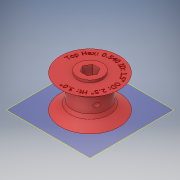
# Autodesk Inventor part: spoolV08upper
Saved by Autodesk Inventor 2019.4 (Build 234330000, 330)
## iProperties
Created: 2019-02-25
Part Number: spoolV08upper
Material: PC/ABS Plastic
Document SubType Name: Modeling
Designer: steele
Density: 0.357273 g/cm^3
Appearance: Smooth - Red
holeForString: 0.200 in
stringDiameter: 0.120 in
clearanceForString: 0.080 in
clearanceForHexShaft: 0.040 in
spoolInteriorDiameter: 1.500 in
spoolInteriroRadius: 0.750 in
spoolExteriorDiameter: 2.500 in
spoolExteriorRadius: 1.250 in
hexHoleChamfer: 0.063 in
stringHoleCenterFromHexShaft: 0.370 in
textCircleDiameter: 1.875 in
textHeight: 0.180 in
textDepth: 0.050 in
Author: steele
Autodesk Inventor part; units mm, degrees
(part 1 of 2)
ref_plane "XZ Plane" through (0, 0, 0) normal (0, 1, 0) x (-1, 0, 0)
sketch "Sketch15" plane through (0, 0, 0) normal (0, 0, 1) x (1, 0, 0)
  line L0 (31.75, 0) -> (31.75, 69.85) construction
  line L1 (12.065, 0) -> (31.75, 0)
  line L2 (13.335, 69.85) -> (31.75, 69.85)
  line L3 (19.05, 0) -> (19.05, 69.85) construction
  line L4 (0, 69.85) -> (0, 0)
  line L5 (19.05, 17.4625) -> (31.75, 17.4625) construction
  line L6 (31.75, 0) -> (19.05, 7.3323)
  line L7 (31.75, 34.925) -> (19.05, 27.5927)
  line L8 (19.05, 27.5927) -> (31.75, 27.5927) construction
  line L9 (19.05, 27.5927) -> (19.05, 7.3323)
  line L10 (31.75, 34.925) -> (19.05, 42.2573)
  line L11 (19.05, 42.2573) -> (19.05, 62.5177)
  line L12 (19.05, 62.5177) -> (31.75, 69.85)
  line L13 (31.75, 34.925) -> (19.05, 34.925) construction
  line L14 (19.05, 62.5177) -> (31.75, 62.5177) construction
  line L15 (0, 69.85) -> (0, 72.39)
  line L16 (0, 72.39) -> (13.335, 72.39)
  line L17 (13.335, 72.39) -> (13.335, 69.85)
  line L18 (0, 0) -> (0, -2.54)
  line L19 (0, -2.54) -> (12.065, -2.54)
  line L20 (12.065, -2.54) -> (12.065, 0)
  dimension "d85" = 31.75
  dimension "d86" = 69.85
  dimension "d87" = 19.05
  dimension "d88" = 31.75
  dimension "d89" = 34.925
  dimension "centerLineForSpool" = 17.4625
  dimension "d93" = 30
  dimension "d94" = 30
  dimension "d95" = 30
  dimension "d96" = 30
  dimension "d149" = 2.54
  dimension "d150" = 13.335
  dimension "d151" = 2.54
  dimension "d152" = 12.065
  constraints: 42 end point, 10 point on line, 5 perpendicular, 3 horizontal, 3 vertical, 2 midpoint, 1 collinear, 1 parallel
  measures "d85" distance from line of L4.end L0
  measures "d86" distance of L0.start L0.end
  measures "d87" distance from line of L3 L4.end
  measures "d88" distance of L4.start L0.end
  measures "d89" distance from line of L7.start L1
  measures "centerLineForSpool" distance from line of L5.start L1
  measures "d93" angle of L6 L1
  measures "d94" angle of L7 L8
  measures "d95" angle of L10 L13
  measures "d96" angle of L12 L14
  measures "d149" distance between parallel lines of L16 L2
  measures "d150" distance between parallel lines of L17 L15
  measures "d151" distance from line of L4.end L19
  measures "d152" distance between parallel lines of L20 L18
revolve "Revolution2" add sketch "Sketch15" angle 360 about axis through (0, 69.85, 0) along (0, -1, 0)
sketch "Sketch16" plane through (0, 0, 0) normal (0, -1, 0) x (1, 0, 0)
  line L0 (-7.9189, 0) -> (-3.9595, 6.858)
  line L1 (-3.9595, 6.858) -> (3.9595, 6.858)
  line L2 (3.9595, 6.858) -> (7.9189, 0)
  line L3 (7.9189, 0) -> (3.9595, -6.858)
  line L4 (3.9595, -6.858) -> (-3.9595, -6.858)
  line L5 (-3.9595, -6.858) -> (-7.9189, 0)
  point P0 (0, 0)
  point P1 (0, 0)
  dimension "d103" = 13.716
  constraints: 12 end point, 1 coincident, 1 horizontal, 13 other
  measures "d103" distance between parallel lines of L1 L4
extrude "Extrusion11" cut sketch "Sketch16" against normal through all
sketch "Sketch17" plane through (0, 0, 0) normal (1, 0, 0) x (0, 1, 0)
  circle A0 centre (52.3875, 9.398) radius 2.54
  circle A1 centre (17.4625, 9.398) radius 2.54
  line L0 (0, 31.75) -> (0, -31.75) projected
  line L1 (69.85, 31.75) -> (69.85, -31.75) projected
  line L2 (0, 6.858) -> (72.39, 6.858) projected
  point P0 (0, 0)
  point P1 (69.85, 6.858)
  dimension "d110" = 17.4625
  dimension "d111" = 17.4625
  dimension "d112" = 5.08
  constraints: 2 centre point, 2 tangent, 1 equal radius
  measures "d110" distance from line of A1.centre L0
  measures "d111" distance from line of A0.centre L1
  measures "d112" diameter of A0
extrude "Extrusion13" cut sketch "Sketch17" along normal through all both and the other way through all
ref_plane "Work Plane4" through (-19.05, 0, 0) normal (1, 0, 0) x (0, 1, 0)
sketch "Sketch22" plane through (-19.05, 0, 0) normal (1, 0, 0) x (0, 1, 0)
  spline S0 degree 7 poles (54.9275, 9.398) (54.9275, 9.7003) (54.8855, 9.9947) (54.8055, 10.2759) (54.6914, 10.5396) (54.547, 10.7823) (54.3764, 11.0012) (53.983, 11.3946) (53.7559, 11.5694) (53.5066, 11.7139) (53.24, 11.8248) (52.9612, 11.9) (52.6753, 11.938) (52.1137, 11.938) (51.8403, 11.9036) (51.5721, 11.8349) (51.3141, 11.7328) (51.0711, 11.5991) (50.848, 11.4367) (50.4419, 11.0554) (50.2585, 10.8324) (50.103, 10.5833) (49.9797, 10.311) (49.8931, 10.0193) (49.8475, 9.713) (49.8475, 9.1243) (49.8819, 8.8508) (49.9506, 8.5825) (50.0528, 8.3245) (50.1864, 8.0817) (50.3487, 7.8586) (50.7502, 7.431) (50.9916, 7.2397) (51.2531, 7.0865) (51.5286, 6.9719) (51.8128, 6.8958) (52.1007, 6.858) (52.7051, 6.858) (53.0247, 6.9043) (53.3394, 6.998) (53.642, 7.1395) (53.9245, 7.3282) (54.1787, 7.563) (54.5393, 8.0279) (54.6661, 8.2331) (54.7705, 8.4538) (54.8497, 8.6855) (54.9021, 8.9235) (54.9275, 9.1626) (54.9275, 9.398) knots 0 0 0 0 0 0 0 0 0.127217 0.127217 0.127217 0.127217 0.127217 0.127217 0.25952 0.25952 0.25952 0.25952 0.25952 0.25952 0.385403 0.385403 0.385403 0.385403 0.385403 0.385403 0.516079 0.516079 0.516079 0.516079 0.516079 0.516079 0.629606 0.629606 0.629606 0.629606 0.629606 0.629606 0.75956 0.75956 0.75956 0.75956 0.75956 0.75956 0.903464 0.903464 0.903464 0.903464 0.903464 0.903464 1 1 1 1 1 1 1 1 projected
  circle A0 centre (52.3875, 9.398) radius 4.7625
  circle A1 centre (52.3875, 9.398) radius 2.54 construction
  line L0 (52.3875, 6.858) -> (72.39, 6.858) construction
  line L1 (69.85, 31.75) -> (69.85, -31.75) construction
  point P0 (0, 0)
  point P1 (69.85, 6.858)
  dimension "d121" = 17.4625
  dimension "d122" = 5.08
  dimension "d125" = 9.525
  constraints: 2 centre point, 1 concentric, 1 tangent, 1 vertical alignment
  measures "d121" distance from line of A1.centre L1
  measures "d122" diameter of A1
  measures "d125" diameter of A0
extrude "Extrusion16" cut sketch "Sketch22" along normal blind 11.1125
ref_plane "Work Plane5" through (19.05, 0, 0) normal (1, 0, 0) x (0, 1, 0)
sketch "Sketch23" plane through (19.05, 0, 0) normal (1, 0, 0) x (0, 1, 0)
  line L0 (17.4625, 6.858) -> (52.3875, 6.858) projected
  circle A0 centre (17.4625, 9.398) radius 2.54 construction
  line L1 (0, 31.75) -> (0, -31.75) projected
  circle A1 centre (17.4625, 9.398) radius 4.7625
  point P0 (0, 0)
  dimension "d127" = 5.08
  dimension "d128" = 17.4625
  dimension "d129" = 9.525
  constraints: 2 centre point, 1 coincident, 1 tangent
  measures "d127" diameter of A0
  measures "d128" distance from line of A0.centre L1
  measures "d129" diameter of A1
extrude "Extrusion17" cut sketch "Sketch23" against normal blind 11.1125
chamfer "Chamfer12" distance 2.3813 angle 45 4 edges at (-19.05, 62.5177, 0) (-19.05, 42.2573, 0) (-19.05, 27.5927, 0) (-19.05, 7.3323, 0)
ref_plane "Work Plane6" through (0, 34.925, 0) normal (0, -1, 0) x (1, 0, 0)
sketch "Sketch24" plane through (0, 69.85, 0) normal (0, 1, 0) x (1, 0, 0)
  circle A0 centre (0, 0) radius 23.8125 construction
  line L0 (-23.7656, 1.5256) -> (-27.7847, 1.8358)
  line L1 (-27.7847, 1.8358) -> (-27.9027, 0.3065)
  line L2 (-27.9027, 0.3065) -> (-28.442, 0.3481)
  line L3 (-28.442, 0.3481) -> (-28.1592, 4.0126)
  line L4 (-28.1592, 4.0126) -> (-27.6199, 3.971)
  line L5 (-27.6199, 3.971) -> (-27.7379, 2.4416)
  line L6 (-27.7379, 2.4416) -> (-23.7188, 2.1315)
  line L7 (-23.7188, 2.1315) -> (-23.7656, 1.5256)
  spline S0 degree 2 poles (-24.5386, 7.2028) (-23.6936, 7.0089) (-22.9592, 5.9851) (-23.115, 5.3062) knots 0 0 0 1 2 2 2
  spline S1 degree 2 poles (-23.115, 5.3062) (-23.2749, 4.6092) (-24.4078, 4.0291) (-25.2239, 4.2164) knots 0 0 0 1 2 2 2
  spline S2 degree 2 poles (-25.2239, 4.2164) (-26.0617, 4.4086) (-26.8008, 5.445) (-26.6467, 6.1166) knots 0 0 0 1 2 2 2
  spline S3 degree 2 poles (-26.6467, 6.1166) (-26.4909, 6.7955) (-25.38, 7.3959) (-24.5386, 7.2028) knots 0 0 0 1 2 2 2
  spline S4 degree 2 poles (-24.672, 6.6214) (-25.322, 6.7706) (-26.0625, 6.4425) (-26.1628, 6.0056) knots 0 0 0 1 2 2 2
  spline S5 degree 2 poles (-26.1628, 6.0056) (-26.263, 5.5686) (-25.7405, 4.9469) (-25.0905, 4.7978) knots 0 0 0 1 2 2 2
  spline S6 degree 2 poles (-25.0905, 4.7978) (-24.4585, 4.6528) (-23.6991, 4.9803) (-23.5988, 5.4172) knots 0 0 0 1 2 2 2
  spline S7 degree 2 poles (-23.5988, 5.4172) (-23.4994, 5.8506) (-24.0292, 6.4739) (-24.672, 6.6214) knots 0 0 0 1 2 2 2
  spline S8 degree 2 poles (-23.3247, 10.7142) (-22.5233, 10.4034) (-21.8728, 9.2729) (-22.0992, 8.6892) knots 0 0 0 1 2 2 2
  spline S9 degree 2 poles (-22.0992, 8.6892) (-22.1916, 8.4508) (-22.4442, 8.1275) (-22.6318, 7.9817) knots 0 0 0 1 2 2 2
  line L8 (-22.6318, 7.9817) -> (-21.2915, 7.462)
  line L9 (-21.2915, 7.462) -> (-21.5005, 6.9231)
  line L10 (-21.5005, 6.9231) -> (-25.8772, 8.6203)
  line L11 (-25.8772, 8.6203) -> (-25.6682, 9.1592)
  line L12 (-25.6682, 9.1592) -> (-25.3332, 9.0293)
  spline S10 degree 2 poles (-25.3332, 9.0293) (-25.4385, 9.3006) (-25.4901, 9.8849) (-25.3789, 10.1716) knots 0 0 0 1 2 2 2
  spline S11 degree 2 poles (-25.3789, 10.1716) (-25.1659, 10.7209) (-24.057, 10.9982) (-23.3247, 10.7142) knots 0 0 0 1 2 2 2
  spline S12 degree 2 poles (-23.4782, 10.1339) (-24.0274, 10.3469) (-24.7672, 10.2325) (-24.9186, 9.8421) knots 0 0 0 1 2 2 2
  spline S13 degree 2 poles (-24.9186, 9.8421) (-25.007, 9.6141) (-24.9693, 9.1067) (-24.8841, 8.8551) knots 0 0 0 1 2 2 2
  line L13 (-24.8841, 8.8551) -> (-23.0671, 8.1505)
  spline S14 degree 2 poles (-23.0671, 8.1505) (-22.8852, 8.3224) (-22.6927, 8.5934) (-22.6176, 8.7869) knots 0 0 0 1 2 2 2
  spline S15 degree 2 poles (-22.6176, 8.7869) (-22.4555, 9.2049) (-22.8909, 9.9062) (-23.4782, 10.1339) knots 0 0 0 1 2 2 2
  line L14 (-18.505, 15.0783) -> (-18.8552, 14.5817)
  line L15 (-18.8552, 14.5817) -> (-20.6841, 15.8712)
  line L16 (-20.6841, 15.8712) -> (-21.8968, 14.1513)
  line L17 (-21.8968, 14.1513) -> (-20.0678, 12.8617)
  line L18 (-20.0678, 12.8617) -> (-20.418, 12.3651)
  line L19 (-20.418, 12.3651) -> (-24.1546, 14.9997)
  line L20 (-24.1546, 14.9997) -> (-23.8045, 15.4963)
  line L21 (-23.8045, 15.4963) -> (-22.3389, 14.463)
  line L22 (-22.3389, 14.463) -> (-21.1262, 16.1829)
  line L23 (-21.1262, 16.1829) -> (-22.5918, 17.2162)
  line L24 (-22.5918, 17.2162) -> (-22.2416, 17.7128)
  line L25 (-22.2416, 17.7128) -> (-18.505, 15.0783)
  spline S16 degree 2 poles (-16.8226, 16.7452) (-17.3966, 16.156) (-18.6882, 16.1523) (-19.2986, 16.747) knots 0 0 0 1 2 2 2
  spline S17 degree 2 poles (-19.2986, 16.747) (-19.8983, 17.3314) (-19.9967, 18.6532) (-19.5029, 19.1601) knots 0 0 0 1 2 2 2
  spline S18 degree 2 poles (-19.5029, 19.1601) (-19.2805, 19.3883) (-18.804, 19.612) (-18.5366, 19.6049) knots 0 0 0 1 2 2 2
  spline S19 degree 2 poles (-18.5366, 19.6049) (-18.2667, 19.6006) (-17.7237, 19.3456) (-17.4291, 19.0586) knots 0 0 0 1 2 2 2
  line L26 (-17.4291, 19.0586) -> (-17.2035, 18.8389)
  line L27 (-17.2035, 18.8389) -> (-18.8609, 17.1379)
  spline S20 degree 2 poles (-18.8609, 17.1379) (-18.4336, 16.7216) (-17.561, 16.7094) (-17.1887, 17.0915) knots 0 0 0 1 2 2 2
  spline S21 degree 2 poles (-17.1887, 17.0915) (-17.0568, 17.2268) (-16.8619, 17.549) (-16.8062, 17.7017) knots 0 0 0 1 2 2 2
  spline S22 degree 2 poles (-16.8062, 17.7017) (-16.7507, 17.8649) (-16.6936, 18.1093) (-16.6869, 18.2011) knots 0 0 0 1 2 2 2
  line L28 (-16.6869, 18.2011) -> (-16.6637, 18.2249)
  line L29 (-16.6637, 18.2249) -> (-16.2126, 17.7854)
  spline S23 degree 2 poles (-16.2126, 17.7854) (-16.2532, 17.6853) (-16.3803, 17.385) (-16.4391, 17.2768) knots 0 0 0 1 2 2 2
  spline S24 degree 2 poles (-16.4391, 17.2768) (-16.521, 17.1237) (-16.6778, 16.8938) (-16.8226, 16.7452) knots 0 0 0 1 2 2 2
  spline S25 degree 2 poles (-17.9123, 18.7432) (-18.0847, 18.9008) (-18.396, 19.0697) (-18.5429, 19.0835) knots 0 0 0 1 2 2 2
  spline S26 degree 2 poles (-18.5429, 19.0835) (-18.7056, 19.1023) (-19.0236, 18.9724) (-19.1865, 18.8052) knots 0 0 0 1 2 2 2
  spline S27 degree 2 poles (-19.1865, 18.8052) (-19.3468, 18.6407) (-19.4736, 18.3142) (-19.4711, 18.1256) knots 0 0 0 1 2 2 2
  spline S28 degree 2 poles (-19.4711, 18.1256) (-19.4634, 17.937) (-19.3203, 17.6114) (-19.1767, 17.4455) knots 0 0 0 1 2 2 2
  line L30 (-19.1767, 17.4455) -> (-17.9123, 18.7432)
  line L31 (-13.4685, 19.6968) -> (-14.0259, 19.2608)
  line L32 (-14.0259, 19.2608) -> (-15.4769, 19.7628)
  line L33 (-15.4769, 19.7628) -> (-15.3567, 18.2199)
  line L34 (-15.3567, 18.2199) -> (-15.8732, 17.8159)
  line L35 (-15.8732, 17.8159) -> (-15.9842, 19.8881)
  line L36 (-15.9842, 19.8881) -> (-17.9782, 20.5251)
  line L37 (-17.9782, 20.5251) -> (-17.4208, 20.9611)
  line L38 (-17.4208, 20.9611) -> (-15.9796, 20.4656)
  line L39 (-15.9796, 20.4656) -> (-16.0988, 21.9951)
  line L40 (-16.0988, 21.9951) -> (-15.5823, 22.3992)
  line L41 (-15.5823, 22.3992) -> (-15.4701, 20.3373)
  line L42 (-15.4701, 20.3373) -> (-13.4685, 19.6968)
  line L43 (-12.1723, 20.4696) -> (-12.797, 20.085)
  line L44 (-12.797, 20.085) -> (-13.2555, 20.8295)
  line L45 (-13.2555, 20.8295) -> (-12.6308, 21.2142)
  line L46 (-12.6308, 21.2142) -> (-12.1723, 20.4696)
  line L47 (-13.5127, 22.6465) -> (-14.1374, 22.2619)
  line L48 (-14.1374, 22.2619) -> (-14.5958, 23.0065)
  line L49 (-14.5958, 23.0065) -> (-13.9711, 23.3911)
  line L50 (-13.9711, 23.3911) -> (-13.5127, 22.6465)
  spline S29 degree 2 poles (-7.5971, 25.0112) (-7.1742, 23.856) (-7.4496, 22.5282) (-8.149, 22.2722) knots 0 0 0 1 2 2 2
  spline S30 degree 2 poles (-8.149, 22.2722) (-8.8587, 22.0124) (-9.927, 22.8721) (-10.3409, 24.0028) knots 0 0 0 1 2 2 2
  spline S31 degree 2 poles (-10.3409, 24.0028) (-10.7663, 25.1649) (-10.4884, 26.4858) (-9.7855, 26.743) knots 0 0 0 1 2 2 2
  spline S32 degree 2 poles (-9.7855, 26.743) (-9.0793, 27.0016) (-8.0072, 26.1315) (-7.5971, 25.0112) knots 0 0 0 1 2 2 2
  spline S33 degree 2 poles (-7.8558, 23.433) (-7.85, 23.6758) (-8.0198, 24.3553) (-8.1816, 24.7972) knots 0 0 0 1 2 2 2
  spline S34 degree 2 poles (-8.1816, 24.7972) (-8.3433, 25.2391) (-8.6511, 25.8642) (-8.8183, 26.0516) knots 0 0 0 1 2 2 2
  spline S35 degree 2 poles (-8.8183, 26.0516) (-8.9855, 26.2389) (-9.371, 26.3543) (-9.6111, 26.2664) knots 0 0 0 1 2 2 2
  spline S36 degree 2 poles (-9.6111, 26.2664) (-9.8511, 26.1785) (-10.078, 25.839) (-10.0857, 25.5797) knots 0 0 0 1 2 2 2
  spline S37 degree 2 poles (-10.0857, 25.5797) (-10.0924, 25.3287) (-9.9105, 24.6378) (-9.7564, 24.2168) knots 0 0 0 1 2 2 2
  spline S38 degree 2 poles (-9.7564, 24.2168) (-9.5908, 23.7645) (-9.3136, 23.1795) (-9.1365, 22.976) knots 0 0 0 1 2 2 2
  spline S39 degree 2 poles (-9.1365, 22.976) (-8.9715, 22.7839) (-8.574, 22.6572) (-8.3234, 22.7489) knots 0 0 0 1 2 2 2
  spline S40 degree 2 poles (-8.3234, 22.7489) (-8.0869, 22.8355) (-7.86, 23.175) (-7.8558, 23.433) knots 0 0 0 1 2 2 2
  line L51 (-5.285, 23.2214) -> (-5.9978, 23.0478)
  line L52 (-5.9978, 23.0478) -> (-6.2048, 23.8973)
  line L53 (-6.2048, 23.8973) -> (-5.492, 24.071)
  line L54 (-5.492, 24.071) -> (-5.285, 23.2214)
  spline S41 degree 2 poles (-1.8255, 25.2371) (-1.7837, 24.91) (-1.9218, 24.3246) (-2.0866, 24.0944) knots 0 0 0 1 2 2 2
  spline S42 degree 2 poles (-2.0866, 24.0944) (-2.2514, 23.8641) (-2.7905, 23.5524) (-3.1433, 23.5073) knots 0 0 0 1 2 2 2
  spline S43 degree 2 poles (-3.1433, 23.5073) (-3.4667, 23.466) (-4.1172, 23.5285) (-4.3632, 23.6129) knots 0 0 0 1 2 2 2
  line L55 (-4.3632, 23.6129) -> (-4.4455, 24.256)
  line L56 (-4.4455, 24.256) -> (-4.4014, 24.2616)
  spline S44 degree 2 poles (-4.4014, 24.2616) (-4.325, 24.2191) (-4.0471, 24.1202) (-3.8816, 24.0816) knots 0 0 0 1 2 2 2
  spline S45 degree 2 poles (-3.8816, 24.0816) (-3.6935, 24.0421) (-3.3869, 24.0103) (-3.1995, 24.0343) knots 0 0 0 1 2 2 2
  spline S46 degree 2 poles (-3.1995, 24.0343) (-3.0157, 24.0578) (-2.6872, 24.2343) (-2.5805, 24.3936) knots 0 0 0 1 2 2 2
  spline S47 degree 2 poles (-2.5805, 24.3936) (-2.484, 24.5441) (-2.4124, 24.9193) (-2.4434, 25.1619) knots 0 0 0 1 2 2 2
  spline S48 degree 2 poles (-2.4434, 25.1619) (-2.4744, 25.4044) (-2.6462, 25.6962) (-2.7843, 25.7831) knots 0 0 0 1 2 2 2
  spline S49 degree 2 poles (-2.7843, 25.7831) (-2.9275, 25.8806) (-3.3219, 25.9273) (-3.5535, 25.8977) knots 0 0 0 1 2 2 2
  spline S50 degree 2 poles (-3.5535, 25.8977) (-3.8034, 25.8658) (-4.2896, 25.7252) (-4.4361, 25.6728) knots 0 0 0 1 2 2 2
  line L57 (-4.4361, 25.6728) -> (-4.7349, 28.0102)
  line L58 (-4.7349, 28.0102) -> (-2.2468, 28.3283)
  line L59 (-2.2468, 28.3283) -> (-2.1787, 27.7954)
  line L60 (-2.1787, 27.7954) -> (-4.0824, 27.552)
  line L61 (-4.0824, 27.552) -> (-3.9279, 26.3429)
  spline S51 degree 2 poles (-3.9279, 26.3429) (-3.8195, 26.3717) (-3.6077, 26.41) (-3.5195, 26.4212) knots 0 0 0 1 2 2 2
  spline S52 degree 2 poles (-3.5195, 26.4212) (-3.1704, 26.4659) (-2.6744, 26.4135) (-2.4323, 26.2726) knots 0 0 0 1 2 2 2
  spline S53 degree 2 poles (-2.4323, 26.2726) (-2.1865, 26.1322) (-1.8782, 25.6487) (-1.8255, 25.2371) knots 0 0 0 1 2 2 2
  line L62 (1.983, 25.3539) -> (1.4385, 25.363)
  line L63 (1.4385, 25.363) -> (1.4123, 23.7923)
  line L64 (1.4123, 23.7923) -> (0.8232, 23.8021)
  line L65 (0.8232, 23.8021) -> (0.8495, 25.3728)
  line L66 (0.8495, 25.3728) -> (-1.1695, 25.4065)
  line L67 (-1.1695, 25.4065) -> (-1.1587, 26.0511)
  line L68 (-1.1587, 26.0511) -> (0.9254, 28.373)
  line L69 (0.9254, 28.373) -> (1.4885, 28.3636)
  line L70 (1.4885, 28.3636) -> (1.4467, 25.8557)
  line L71 (1.4467, 25.8557) -> (1.9913, 25.8466)
  line L72 (1.9913, 25.8466) -> (1.983, 25.3539)
  line L73 (0.8577, 25.8655) -> (0.8875, 27.6511)
  line L74 (0.8875, 27.6511) -> (-0.6797, 25.8911)
  line L75 (-0.6797, 25.8911) -> (0.8577, 25.8655)
  spline S54 degree 2 poles (5.6158, 25.5291) (5.4192, 24.3149) (4.5292, 23.2917) (3.7941, 23.4107) knots 0 0 0 1 2 2 2
  spline S55 degree 2 poles (3.7941, 23.4107) (3.0479, 23.5315) (2.5371, 24.804) (2.7295, 25.9927) knots 0 0 0 1 2 2 2
  spline S56 degree 2 poles (2.7295, 25.9927) (2.9273, 27.2142) (3.8162, 28.2301) (4.555, 28.1105) knots 0 0 0 1 2 2 2
  spline S57 degree 2 poles (4.555, 28.1105) (5.2974, 27.9903) (5.8065, 26.7068) (5.6158, 25.5291) knots 0 0 0 1 2 2 2
  spline S58 degree 2 poles (4.6178, 24.2795) (4.7417, 24.4884) (4.9262, 25.1641) (5.0014, 25.6286) knots 0 0 0 1 2 2 2
  spline S59 degree 2 poles (5.0014, 25.6286) (5.0766, 26.0931) (5.1142, 26.7889) (5.06, 27.0341) knots 0 0 0 1 2 2 2
  spline S60 degree 2 poles (5.06, 27.0341) (5.0059, 27.2793) (4.7262, 27.5686) (4.4738, 27.6094) knots 0 0 0 1 2 2 2
  spline S61 degree 2 poles (4.4738, 27.6094) (4.2215, 27.6503) (3.8575, 27.4652) (3.7239, 27.2429) knots 0 0 0 1 2 2 2
  spline S62 degree 2 poles (3.7239, 27.2429) (3.5952, 27.0273) (3.4156, 26.3357) (3.344, 25.8932) knots 0 0 0 1 2 2 2
  spline S63 degree 2 poles (3.344, 25.8932) (3.267, 25.4177) (3.2225, 24.7719) (3.2773, 24.5078) knots 0 0 0 1 2 2 2
  spline S64 degree 2 poles (3.2773, 24.5078) (3.3272, 24.2595) (3.6118, 23.9544) (3.8752, 23.9118) knots 0 0 0 1 2 2 2
  spline S65 degree 2 poles (3.8752, 23.9118) (4.1239, 23.8715) (4.4879, 24.0565) (4.6178, 24.2795) knots 0 0 0 1 2 2 2
  line L76 (9.3044, 21.9373) -> (7.6495, 22.5679)
  line L77 (7.6495, 22.5679) -> (7.8157, 23.0041)
  line L78 (7.8157, 23.0041) -> (8.3593, 22.797)
  line L79 (8.3593, 22.797) -> (9.6547, 26.1969)
  line L80 (9.6547, 26.1969) -> (9.1112, 26.404)
  line L81 (9.1112, 26.404) -> (9.2774, 26.8402)
  line L82 (9.2774, 26.8402) -> (10.9323, 26.2096)
  line L83 (10.9323, 26.2096) -> (10.7661, 25.7734)
  line L84 (10.7661, 25.7734) -> (10.2225, 25.9805)
  line L85 (10.2225, 25.9805) -> (8.9271, 22.5806)
  line L86 (8.9271, 22.5806) -> (9.4706, 22.3735)
  line L87 (9.4706, 22.3735) -> (9.3044, 21.9373)
  spline S66 degree 2 poles (14.2656, 21.9358) (13.964, 21.3871) (13.0337, 20.7484) (12.5247, 20.7069) knots 0 0 0 1 2 2 2
  spline S67 degree 2 poles (12.5247, 20.7069) (12.1142, 20.6831) (11.4162, 20.8976) (10.9291, 21.1653) knots 0 0 0 1 2 2 2
  line L88 (10.9291, 21.1653) -> (10.007, 21.6721)
  line L89 (10.007, 21.6721) -> (12.2092, 25.6788)
  line L90 (12.2092, 25.6788) -> (13.1216, 25.1773)
  spline S68 degree 2 poles (13.1216, 25.1773) (13.6865, 24.8668) (14.2366, 24.3446) (14.3818, 24.0704) knots 0 0 0 1 2 2 2
  spline S69 degree 2 poles (14.3818, 24.0704) (14.6272, 23.6015) (14.5868, 22.5203) (14.2656, 21.9358) knots 0 0 0 1 2 2 2
  spline S70 degree 2 poles (13.7139, 22.2475) (13.9673, 22.7085) (14.0208, 23.5289) (13.8206, 23.88) knots 0 0 0 1 2 2 2
  spline S71 degree 2 poles (13.8206, 23.88) (13.6759, 24.1244) (13.2545, 24.5039) (12.8941, 24.702) knots 0 0 0 1 2 2 2
  line L91 (12.8941, 24.702) -> (12.4883, 24.9251)
  line L92 (12.4883, 24.9251) -> (10.7929, 21.8405)
  line L93 (10.7929, 21.8405) -> (11.1988, 21.6174)
  spline S72 degree 2 poles (11.1988, 21.6174) (11.5527, 21.4229) (12.1509, 21.2421) (12.4523, 21.2751) knots 0 0 0 1 2 2 2
  spline S73 degree 2 poles (12.4523, 21.2751) (12.835, 21.31) (13.4569, 21.7799) (13.7139, 22.2475) knots 0 0 0 1 2 2 2
  line L94 (16.0104, 20.9553) -> (15.4213, 21.3925)
  line L95 (15.4213, 21.3925) -> (15.9424, 22.0947)
  line L96 (15.9424, 22.0947) -> (16.5315, 21.6574)
  line L97 (16.5315, 21.6574) -> (16.0104, 20.9553)
  line L98 (14.4867, 18.9025) -> (13.8976, 19.3397)
  line L99 (13.8976, 19.3397) -> (14.4188, 20.0419)
  line L100 (14.4188, 20.0419) -> (15.0078, 19.6046)
  line L101 (15.0078, 19.6046) -> (14.4867, 18.9025)
  line L102 (18.5302, 15.0042) -> (17.0406, 16.6643)
  line L103 (17.0406, 16.6643) -> (17.3881, 16.976)
  line L104 (17.3881, 16.976) -> (17.9424, 16.3583)
  line L105 (17.9424, 16.3583) -> (20.2229, 18.4046)
  line L106 (20.2229, 18.4046) -> (19.6687, 19.0224)
  line L107 (19.6687, 19.0224) -> (19.9803, 19.302)
  spline S74 degree 2 poles (19.9803, 19.302) (20.2945, 18.9517) (20.79, 18.799) (21.0856, 19.0244) knots 0 0 0 1 2 2 2
  line L108 (21.0856, 19.0244) -> (21.4023, 18.6714)
  line L109 (21.4023, 18.6714) -> (18.3358, 15.9199)
  line L110 (18.3358, 15.9199) -> (18.8777, 15.3159)
  line L111 (18.8777, 15.3159) -> (18.5302, 15.0042)
  line L112 (19.5991, 13.5293) -> (19.1732, 14.1266)
  line L113 (19.1732, 14.1266) -> (19.8851, 14.6342)
  line L114 (19.8851, 14.6342) -> (20.311, 14.037)
  line L115 (20.311, 14.037) -> (19.5991, 13.5293)
  spline S75 degree 2 poles (22.7552, 11.0655) (22.467, 10.9053) (21.8722, 10.8161) (21.5972, 10.8836) knots 0 0 0 1 2 2 2
  spline S76 degree 2 poles (21.5972, 10.8836) (21.3223, 10.9512) (20.8327, 11.336) (20.6598, 11.6468) knots 0 0 0 1 2 2 2
  spline S77 degree 2 poles (20.6598, 11.6468) (20.5013, 11.9318) (20.3179, 12.5589) (20.3048, 12.8188) knots 0 0 0 1 2 2 2
  line L116 (20.3048, 12.8188) -> (20.8714, 13.1339)
  line L117 (20.8714, 13.1339) -> (20.893, 13.095)
  spline S78 degree 2 poles (20.893, 13.095) (20.8819, 13.0083) (20.8932, 12.7136) (20.9188, 12.5455) knots 0 0 0 1 2 2 2
  spline S79 degree 2 poles (20.9188, 12.5455) (20.952, 12.3563) (21.0364, 12.0598) (21.1282, 11.8946) knots 0 0 0 1 2 2 2
  spline S80 degree 2 poles (21.1282, 11.8946) (21.2183, 11.7327) (21.5041, 11.4932) (21.6916, 11.4533) knots 0 0 0 1 2 2 2
  spline S81 degree 2 poles (21.6916, 11.4533) (21.8672, 11.4196) (22.2422, 11.4925) (22.4559, 11.6113) knots 0 0 0 1 2 2 2
  spline S82 degree 2 poles (22.4559, 11.6113) (22.6696, 11.7302) (22.8767, 11.998) (22.9062, 12.1585) knots 0 0 0 1 2 2 2
  spline S83 degree 2 poles (22.9062, 12.1585) (22.9435, 12.3277) (22.8404, 12.7112) (22.727, 12.9152) knots 0 0 0 1 2 2 2
  spline S84 degree 2 poles (22.727, 12.9152) (22.6045, 13.1354) (22.2934, 13.5347) (22.1905, 13.6513) knots 0 0 0 1 2 2 2
  line L118 (22.1905, 13.6513) -> (24.2498, 14.7966)
  line L119 (24.2498, 14.7966) -> (25.4689, 12.6045)
  line L120 (25.4689, 12.6045) -> (24.9994, 12.3434)
  line L121 (24.9994, 12.3434) -> (24.0666, 14.0206)
  line L122 (24.0666, 14.0206) -> (23.0013, 13.4282)
  spline S85 degree 2 poles (23.0013, 13.4282) (23.0683, 13.3382) (23.1825, 13.1558) (23.2257, 13.0781) knots 0 0 0 1 2 2 2
  spline S86 degree 2 poles (23.2257, 13.0781) (23.3968, 12.7705) (23.5323, 12.2905) (23.4914, 12.0134) knots 0 0 0 1 2 2 2
  spline S87 degree 2 poles (23.4914, 12.0134) (23.4523, 11.733) (23.1178, 11.2672) (22.7552, 11.0655) knots 0 0 0 1 2 2 2
  line L123 (26.8611, 9.8287) -> (25.1616, 9.2883)
  line L124 (25.1616, 9.2883) -> (25.0108, 9.6629)
  line L125 (25.0108, 9.6629) -> (26.6107, 10.4508)
  line L126 (26.6107, 10.4508) -> (26.8611, 9.8287)
  line L127 (26.4295, 10.901) -> (24.7299, 10.3606)
  line L128 (24.7299, 10.3606) -> (24.5791, 10.7352)
  line L129 (24.5791, 10.7352) -> (26.179, 11.5231)
  line L130 (26.179, 11.5231) -> (26.4295, 10.901)
  spline S88 degree 2 poles (27.7577, 2.8241) (27.4973, 2.5212) (26.6631, 2.099) (26.0992, 2.0114) knots 0 0 0 1 2 2 2
  spline S89 degree 2 poles (26.0992, 2.0114) (25.5501, 1.926) (24.6172, 2.066) (24.276, 2.2829) knots 0 0 0 1 2 2 2
  spline S90 degree 2 poles (24.276, 2.2829) (23.9179, 2.5122) (23.5033, 3.2014) (23.4345, 3.6444) knots 0 0 0 1 2 2 2
  spline S91 degree 2 poles (23.4345, 3.6444) (23.3633, 4.1021) (23.5607, 4.8826) (23.8231, 5.1971) knots 0 0 0 1 2 2 2
  spline S92 degree 2 poles (23.8231, 5.1971) (24.0829, 5.5037) (24.9219, 5.9191) (25.4784, 6.0056) knots 0 0 0 1 2 2 2
  spline S93 degree 2 poles (25.4784, 6.0056) (26.0459, 6.0938) (26.9537, 5.9462) (27.3053, 5.7346) knots 0 0 0 1 2 2 2
  spline S94 degree 2 poles (27.3053, 5.7346) (27.6465, 5.5177) (28.072, 4.8302) (28.1426, 4.3762) knots 0 0 0 1 2 2 2
  spline S95 degree 2 poles (28.1426, 4.3762) (28.2143, 3.9149) (28.0071, 3.1253) (27.7577, 2.8241) knots 0 0 0 1 2 2 2
  spline S96 degree 2 poles (26.0019, 2.6374) (26.4486, 2.7069) (27.1104, 3.0084) (27.31, 3.2195) knots 0 0 0 1 2 2 2
  spline S97 degree 2 poles (27.31, 3.2195) (27.5165, 3.4353) (27.6722, 3.9769) (27.6233, 4.2918) knots 0 0 0 1 2 2 2
  spline S98 degree 2 poles (27.6233, 4.2918) (27.5727, 4.6176) (27.2694, 5.0729) (26.9988, 5.2221) knots 0 0 0 1 2 2 2
  spline S99 degree 2 poles (26.9988, 5.2221) (26.7402, 5.3656) (26.015, 5.4478) (25.5757, 5.3796) knots 0 0 0 1 2 2 2
  spline S100 degree 2 poles (25.5757, 5.3796) (24.6861, 5.2413) (23.8576, 4.3476) (23.9549, 3.7216) knots 0 0 0 1 2 2 2
  spline S101 degree 2 poles (23.9549, 3.7216) (24.0522, 3.0955) (25.1123, 2.4991) (26.0019, 2.6374) knots 0 0 0 1 2 2 2
  spline S102 degree 2 poles (26.0297, -2.6726) (25.4038, -2.6549) (24.4107, -2.119) (24.1413, -1.6852) knots 0 0 0 1 2 2 2
  spline S103 degree 2 poles (24.1413, -1.6852) (23.9326, -1.3309) (23.8047, -0.6119) (23.8204, -0.0563) knots 0 0 0 1 2 2 2
  line L131 (23.8204, -0.0563) -> (23.8502, 0.9955)
  line L132 (23.8502, 0.9955) -> (28.4203, 0.8662)
  line L133 (28.4203, 0.8662) -> (28.3909, -0.1744)
  spline S104 degree 2 poles (28.3909, -0.1744) (28.3727, -0.8189) (28.1594, -1.5467) (27.9817, -1.8012) knots 0 0 0 1 2 2 2
  spline S105 degree 2 poles (27.9817, -1.8012) (27.6766, -2.2336) (26.6963, -2.6914) (26.0297, -2.6726) knots 0 0 0 1 2 2 2
  spline S106 degree 2 poles (26.055, -2.0395) (26.5809, -2.0544) (27.3351, -1.7273) (27.556, -1.3888) knots 0 0 0 1 2 2 2
  spline S107 degree 2 poles (27.556, -1.3888) (27.7073, -1.1485) (27.8525, -0.6003) (27.8642, -0.1892) knots 0 0 0 1 2 2 2
  line L134 (27.8642, -0.1892) -> (27.8773, 0.2737)
  line L135 (27.8773, 0.2737) -> (24.3589, 0.3732)
  line L136 (24.3589, 0.3732) -> (24.3458, -0.0897)
  spline S108 degree 2 poles (24.3458, -0.0897) (24.3344, -0.4934) (24.4467, -1.1082) (24.6138, -1.3612) knots 0 0 0 1 2 2 2
  spline S109 degree 2 poles (24.6138, -1.3612) (24.8196, -1.6858) (25.5217, -2.0244) (26.055, -2.0395) knots 0 0 0 1 2 2 2
  line L137 (23.4322, -4.2547) -> (23.5521, -3.5309)
  line L138 (23.5521, -3.5309) -> (24.4147, -3.6739)
  line L139 (24.4147, -3.6739) -> (24.2948, -4.3976)
  line L140 (24.2948, -4.3976) -> (23.4322, -4.2547)
  line L141 (25.9543, -4.6726) -> (26.0742, -3.9489)
  line L142 (26.0742, -3.9489) -> (26.9368, -4.0918)
  line L143 (26.9368, -4.0918) -> (26.8169, -4.8155)
  line L144 (26.8169, -4.8155) -> (25.9543, -4.6726)
  line L145 (21.7288, -9.8468) -> (22.7358, -7.2132)
  line L146 (22.7358, -7.2132) -> (23.3414, -7.4448)
  spline S110 degree 2 poles (23.3414, -7.4448) (23.4993, -7.8304) (23.801, -8.5249) (23.9749, -8.869) knots 0 0 0 1 2 2 2
  spline S111 degree 2 poles (23.9749, -8.869) (24.3247, -9.5621) (24.8321, -10.1647) (25.1748, -10.2956) knots 0 0 0 1 2 2 2
  spline S112 degree 2 poles (25.1748, -10.2956) (25.3547, -10.3644) (25.667, -10.3569) (25.7919, -10.2896) knots 0 0 0 1 2 2 2
  spline S113 degree 2 poles (25.7919, -10.2896) (25.9168, -10.2223) (26.1038, -9.9924) (26.1647, -9.8332) knots 0 0 0 1 2 2 2
  spline S114 degree 2 poles (26.1647, -9.8332) (26.2229, -9.681) (26.2659, -9.3404) (26.2613, -9.176) knots 0 0 0 1 2 2 2
  spline S115 degree 2 poles (26.2613, -9.176) (26.2592, -9.0363) (26.2067, -8.7585) (26.1847, -8.6707) knots 0 0 0 1 2 2 2
  line L147 (26.1847, -8.6707) -> (26.1967, -8.6396)
  line L148 (26.1967, -8.6396) -> (26.8057, -8.8725)
  spline S116 degree 2 poles (26.8057, -8.8725) (26.8248, -9.082) (26.7522, -9.7802) (26.6437, -10.064) knots 0 0 0 1 2 2 2
  spline S117 degree 2 poles (26.6437, -10.064) (26.4148, -10.6627) (25.5235, -11.0954) (24.9836, -10.889) knots 0 0 0 1 2 2 2
  spline S118 degree 2 poles (24.9836, -10.889) (24.731, -10.7924) (24.3538, -10.5133) (24.2135, -10.3406) knots 0 0 0 1 2 2 2
  spline S119 degree 2 poles (24.2135, -10.3406) (24.0663, -10.1654) (23.8146, -9.724) (23.7016, -9.4904) knots 0 0 0 1 2 2 2
  spline S120 degree 2 poles (23.7016, -9.4904) (23.5107, -9.108) (23.1335, -8.2062) (23.0255, -7.9388) knots 0 0 0 1 2 2 2
  line L149 (23.0255, -7.9388) -> (22.2237, -10.036)
  line L150 (22.2237, -10.036) -> (21.7288, -9.8468)
  line L151 (20.987, -11.2567) -> (21.3238, -10.605)
  line L152 (21.3238, -10.605) -> (22.1006, -11.0065)
  line L153 (22.1006, -11.0065) -> (21.7637, -11.6582)
  line L154 (21.7637, -11.6582) -> (20.987, -11.2567)
  spline S121 degree 2 poles (20.2366, -15.1896) (19.9624, -15.0065) (19.6114, -14.518) (19.5459, -14.2426) knots 0 0 0 1 2 2 2
  spline S122 degree 2 poles (19.5459, -14.2426) (19.4804, -13.9671) (19.5991, -13.3558) (19.7967, -13.0601) knots 0 0 0 1 2 2 2
  spline S123 degree 2 poles (19.7967, -13.0601) (19.9778, -12.789) (20.452, -12.3393) (20.6771, -12.209) knots 0 0 0 1 2 2 2
  line L155 (20.6771, -12.209) -> (21.2163, -12.5692)
  line L156 (21.2163, -12.5692) -> (21.1916, -12.6062)
  spline S124 degree 2 poles (21.1916, -12.6062) (21.1094, -12.6359) (20.8523, -12.7805) (20.7145, -12.8801) knots 0 0 0 1 2 2 2
  spline S125 degree 2 poles (20.7145, -12.8801) (20.5613, -12.996) (20.3361, -13.2065) (20.2311, -13.3636) knots 0 0 0 1 2 2 2
  spline S126 degree 2 poles (20.2311, -13.3636) (20.1282, -13.5177) (20.0456, -13.8813) (20.0958, -14.0664) knots 0 0 0 1 2 2 2
  spline S127 degree 2 poles (20.0958, -14.0664) (20.146, -14.238) (20.3821, -14.5383) (20.5854, -14.6741) knots 0 0 0 1 2 2 2
  spline S128 degree 2 poles (20.5854, -14.6741) (20.7887, -14.81) (21.1216, -14.8719) (21.2779, -14.8248) knots 0 0 0 1 2 2 2
  spline S129 degree 2 poles (21.2779, -14.8248) (21.4454, -14.7808) (21.7395, -14.5139) (21.8692, -14.3198) knots 0 0 0 1 2 2 2
  spline S130 degree 2 poles (21.8692, -14.3198) (22.0092, -14.1103) (22.2223, -13.6512) (22.279, -13.5063) knots 0 0 0 1 2 2 2
  line L157 (22.279, -13.5063) -> (24.2384, -14.8153)
  line L158 (24.2384, -14.8153) -> (22.845, -16.901)
  line L159 (22.845, -16.901) -> (22.3983, -16.6026)
  line L160 (22.3983, -16.6026) -> (23.4644, -15.0067)
  line L161 (23.4644, -15.0067) -> (22.4508, -14.3296)
  spline S131 degree 2 poles (22.4508, -14.3296) (22.4014, -14.4303) (22.2913, -14.6151) (22.2419, -14.6891) knots 0 0 0 1 2 2 2
  spline S132 degree 2 poles (22.2419, -14.6891) (22.0464, -14.9817) (21.6812, -15.3215) (21.416, -15.4117) knots 0 0 0 1 2 2 2
  spline S133 degree 2 poles (21.416, -15.4117) (21.1488, -15.505) (20.5816, -15.4202) (20.2366, -15.1896) knots 0 0 0 1 2 2 2
  line L162 (21.0115, -19.4073) -> (19.7545, -18.1421)
  line L163 (19.7545, -18.1421) -> (20.0189, -17.8368)
  line L164 (20.0189, -17.8368) -> (21.4505, -18.9004)
  line L165 (21.4505, -18.9004) -> (21.0115, -19.4073)
  line L166 (21.7683, -18.5335) -> (20.5113, -17.2683)
  line L167 (20.5113, -17.2683) -> (20.7757, -16.9631)
  line L168 (20.7757, -16.9631) -> (22.2073, -18.0266)
  line L169 (22.2073, -18.0266) -> (21.7683, -18.5335)
  line L170 (12.7431, -20.1842) -> (13.2331, -19.8249)
  line L171 (13.2331, -19.8249) -> (14.5564, -21.6295)
  line L172 (14.5564, -21.6295) -> (16.2535, -20.3851)
  line L173 (16.2535, -20.3851) -> (14.9301, -18.5804)
  line L174 (14.9301, -18.5804) -> (15.4201, -18.2211)
  line L175 (15.4201, -18.2211) -> (18.1238, -21.908)
  line L176 (18.1238, -21.908) -> (17.6338, -22.2674)
  line L177 (17.6338, -22.2674) -> (16.5734, -20.8213)
  line L178 (16.5734, -20.8213) -> (14.8763, -22.0658)
  line L179 (14.8763, -22.0658) -> (15.9368, -23.5118)
  line L180 (15.9368, -23.5118) -> (15.4468, -23.8712)
  line L181 (15.4468, -23.8712) -> (12.7431, -20.1842)
  spline S134 degree 2 poles (11.0228, -21.0363) (11.4358, -20.8108) (12.1582, -21.0285) (12.4369, -21.5391) knots 0 0 0 1 2 2 2
  line L182 (12.4369, -21.5391) -> (13.3476, -23.2074)
  line L183 (13.3476, -23.2074) -> (13.6891, -23.021)
  line L184 (13.6891, -23.021) -> (13.9181, -23.4405)
  line L185 (13.9181, -23.4405) -> (13.5766, -23.6269)
  line L186 (13.5766, -23.6269) -> (14.0488, -24.492)
  line L187 (14.0488, -24.492) -> (13.5415, -24.7689)
  line L188 (13.5415, -24.7689) -> (13.0693, -23.9039)
  line L189 (13.0693, -23.9039) -> (12.1359, -24.4133)
  line L190 (12.1359, -24.4133) -> (11.9069, -23.9938)
  line L191 (11.9069, -23.9938) -> (12.8403, -23.4844)
  line L192 (12.8403, -23.4844) -> (12.0574, -22.0502)
  spline S135 degree 2 poles (12.0574, -22.0502) (11.9332, -21.8225) (11.7802, -21.581) (11.6663, -21.5039) knots 0 0 0 1 2 2 2
  spline S136 degree 2 poles (11.6663, -21.5039) (11.5693, -21.4344) (11.313, -21.4519) (11.1374, -21.5478) knots 0 0 0 1 2 2 2
  spline S137 degree 2 poles (11.1374, -21.5478) (11.0138, -21.6153) (10.8237, -21.8161) (10.7841, -21.8673) knots 0 0 0 1 2 2 2
  line L193 (10.7841, -21.8673) -> (10.7548, -21.8832)
  line L194 (10.7548, -21.8832) -> (10.5063, -21.4279)
  spline S138 degree 2 poles (10.5063, -21.4279) (10.6281, -21.3108) (10.8959, -21.1055) (11.0228, -21.0363) knots 0 0 0 1 2 2 2
  line L195 (10.1467, -24.3414) -> (10.8198, -24.0497)
  line L196 (10.8198, -24.0497) -> (11.1674, -24.852)
  line L197 (11.1674, -24.852) -> (10.4943, -25.1437)
  line L198 (10.4943, -25.1437) -> (10.1467, -24.3414)
  line L199 (9.1303, -21.9956) -> (9.8035, -21.704)
  line L200 (9.8035, -21.704) -> (10.1511, -22.5063)
  line L201 (10.1511, -22.5063) -> (9.478, -22.7979)
  line L202 (9.478, -22.7979) -> (9.1303, -21.9956)
  spline S139 degree 2 poles (5.9137, -27.3187) (6.0769, -27.2842) (6.3827, -27.1364) (6.5256, -27.0419) knots 0 0 0 1 2 2 2
  spline S140 degree 2 poles (6.5256, -27.0419) (6.6576, -26.9497) (6.844, -26.7741) (6.9151, -26.6985) knots 0 0 0 1 2 2 2
  line L203 (6.9151, -26.6985) -> (6.9514, -26.6908)
  line L204 (6.9514, -26.6908) -> (7.0852, -27.3253)
  spline S141 degree 2 poles (7.0852, -27.3253) (6.9116, -27.4717) (6.2768, -27.7835) (5.976, -27.847) knots 0 0 0 1 2 2 2
  spline S142 degree 2 poles (5.976, -27.847) (5.6714, -27.9112) (5.1923, -27.8836) (4.9799, -27.7921) knots 0 0 0 1 2 2 2
  spline S143 degree 2 poles (4.9799, -27.7921) (4.7543, -27.692) (4.4648, -27.3251) (4.4067, -27.0496) knots 0 0 0 1 2 2 2
  spline S144 degree 2 poles (4.4067, -27.0496) (4.3287, -26.6798) (4.6968, -26.0191) (5.0222, -25.8747) knots 0 0 0 1 2 2 2
  line L205 (5.0222, -25.8747) -> (5.0131, -25.8312)
  spline S145 degree 2 poles (5.0131, -25.8312) (4.8656, -25.832) (4.5154, -25.7696) (4.3501, -25.6681) knots 0 0 0 1 2 2 2
  spline S146 degree 2 poles (4.3501, -25.6681) (4.1856, -25.5703) (3.9259, -25.201) (3.864, -24.9073) knots 0 0 0 1 2 2 2
  spline S147 degree 2 poles (3.864, -24.9073) (3.8005, -24.6064) (3.8993, -24.0517) (4.0466, -23.8161) knots 0 0 0 1 2 2 2
  spline S148 degree 2 poles (4.0466, -23.8161) (4.1995, -23.5718) (4.7098, -23.2446) (5.0615, -23.1704) knots 0 0 0 1 2 2 2
  spline S149 degree 2 poles (5.0615, -23.1704) (5.3986, -23.0993) (6.0928, -23.1232) (6.3413, -23.1882) knots 0 0 0 1 2 2 2
  line L206 (6.3413, -23.1882) -> (6.4751, -23.8226)
  line L207 (6.4751, -23.8226) -> (6.4316, -23.8318)
  spline S150 degree 2 poles (6.4316, -23.8318) (6.214, -23.7338) (5.5225, -23.6146) (5.2071, -23.6812) knots 0 0 0 1 2 2 2
  spline S151 degree 2 poles (5.2071, -23.6812) (5.0222, -23.7202) (4.6769, -23.9142) (4.5819, -24.0743) knots 0 0 0 1 2 2 2
  spline S152 degree 2 poles (4.5819, -24.0743) (4.4906, -24.2337) (4.431, -24.5795) (4.4822, -24.8223) knots 0 0 0 1 2 2 2
  spline S153 degree 2 poles (4.4822, -24.8223) (4.5334, -25.0652) (4.7413, -25.3508) (4.8874, -25.4147) knots 0 0 0 1 2 2 2
  spline S154 degree 2 poles (4.8874, -25.4147) (5.0334, -25.4785) (5.3923, -25.4748) (5.5953, -25.432) knots 0 0 0 1 2 2 2
  line L208 (5.5953, -25.432) -> (5.8491, -25.3784)
  line L209 (5.8491, -25.3784) -> (5.9538, -25.8751)
  line L210 (5.9538, -25.8751) -> (5.7544, -25.9172)
  spline S155 degree 2 poles (5.7544, -25.9172) (5.352, -26.002) (4.9255, -26.4934) (5.0028, -26.8595) knots 0 0 0 1 2 2 2
  spline S156 degree 2 poles (5.0028, -26.8595) (5.0387, -27.0299) (5.2205, -27.2453) (5.3409, -27.2956) knots 0 0 0 1 2 2 2
  spline S157 degree 2 poles (5.3409, -27.2956) (5.4693, -27.348) (5.7578, -27.3515) (5.9137, -27.3187) knots 0 0 0 1 2 2 2
  line L211 (1.9211, -23.7377) -> (2.6513, -23.6673)
  line L212 (2.6513, -23.6673) -> (2.7351, -24.5377)
  line L213 (2.7351, -24.5377) -> (2.0049, -24.608)
  line L214 (2.0049, -24.608) -> (1.9211, -23.7377)
  spline S158 degree 2 poles (-1.8777, -26.072) (-1.8582, -24.8421) (-1.1249, -23.7013) (-0.3803, -23.7131) knots 0 0 0 1 2 2 2
  spline S159 degree 2 poles (-0.3803, -23.7131) (0.3754, -23.7251) (1.0644, -24.9107) (1.0452, -26.1147) knots 0 0 0 1 2 2 2
  spline S160 degree 2 poles (1.0452, -26.1147) (1.0256, -27.352) (0.2924, -28.4854) (-0.4559, -28.4735) knots 0 0 0 1 2 2 2
  spline S161 degree 2 poles (-0.4559, -28.4735) (-1.2079, -28.4615) (-1.8967, -27.2648) (-1.8777, -26.072) knots 0 0 0 1 2 2 2
  spline S162 degree 2 poles (-1.0702, -24.6915) (-1.1627, -24.9161) (-1.2479, -25.6114) (-1.2554, -26.0819) knots 0 0 0 1 2 2 2
  spline S163 degree 2 poles (-1.2554, -26.0819) (-1.2628, -26.5523) (-1.1997, -27.2463) (-1.1108, -27.4811) knots 0 0 0 1 2 2 2
  spline S164 degree 2 poles (-1.1108, -27.4811) (-1.0219, -27.716) (-0.7035, -27.9619) (-0.4478, -27.966) knots 0 0 0 1 2 2 2
  spline S165 degree 2 poles (-0.4478, -27.966) (-0.1922, -27.97) (0.1413, -27.7345) (0.2414, -27.4952) knots 0 0 0 1 2 2 2
  spline S166 degree 2 poles (0.2414, -27.4952) (0.3378, -27.2633) (0.4157, -26.5531) (0.4229, -26.1048) knots 0 0 0 1 2 2 2
  spline S167 degree 2 poles (0.4229, -26.1048) (0.4305, -25.6232) (0.3815, -24.9777) (0.2892, -24.7242) knots 0 0 0 1 2 2 2
  spline S168 degree 2 poles (0.2892, -24.7242) (0.204, -24.4857) (-0.1216, -24.2249) (-0.3884, -24.2206) knots 0 0 0 1 2 2 2
  spline S169 degree 2 poles (-0.3884, -24.2206) (-0.6403, -24.2166) (-0.9738, -24.4522) (-1.0702, -24.6915) knots 0 0 0 1 2 2 2
  line L215 (-3.7695, -28.3397) -> (-3.388, -26.5976)
  line L216 (-3.388, -26.5976) -> (-2.9882, -26.6542)
  line L217 (-2.9882, -26.6542) -> (-3.1055, -28.4338)
  line L218 (-3.1055, -28.4338) -> (-3.7695, -28.3397)
  line L219 (-4.9141, -28.1776) -> (-4.5326, -26.4355)
  line L220 (-4.5326, -26.4355) -> (-4.1327, -26.4921)
  line L221 (-4.1327, -26.4921) -> (-4.2501, -28.2716)
  line L222 (-4.2501, -28.2716) -> (-4.9141, -28.1776)
  dimension "d142" = 47.625
  constraints: 1 centre point, 1 coincident, 1 other
  measures "d142" diameter of A0
extrude "Extrusion18" cut sketch "Sketch24" against normal blind 1.27